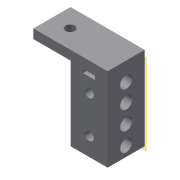
# Autodesk Inventor part: Neje_20mm_rod_connector_double
Saved by Autodesk Inventor 2019.4 (Build 234330000, 330)
## iProperties
Created: 2021-09-21
Part Number: Neje_20mm_rod_connector_double
Material: Generic
Document SubType Name: Modeling
Designer: diederichbenedict
Density: 1 g/cm^3
Appearance: Default
Author: diederichbenedict
Autodesk Inventor part; units mm, degrees
ref_plane "YZ Plane" through (0, 0, 0) normal (1, 0, 0) x (0, 1, 0)
ref_plane "XZ Plane" through (0, 0, 0) normal (0, 1, 0) x (-1, 0, 0)
ref_plane "Work Plane1" through (0, 0, 0) normal (0, 0, 1) x (1, 0, 0)
sketch "Sketch1" plane through (0, 0, 0) normal (0, 0, 1) x (1, 0, 0)
  circle A0 centre (0, 0) radius 2 construction
  circle A1 centre (0, 20) radius 2.5 construction
  line L0 (-10, 4) -> (-10, 16) construction
  line L1 (-10, 4) -> (-6, 4) construction
  line L2 (-6, 4) -> (-6, -4) construction
  line L3 (-6, -4) -> (-10, -4) construction
  line L4 (-10, -4) -> (-10, -10) construction
  line L5 (-10, -10) -> (-4, -10) construction
  line L6 (-4, -10) -> (-4, -6) construction
  line L7 (-4, -6) -> (4, -6) construction
  line L8 (4, -6) -> (4, -10) construction
  line L9 (4, -10) -> (10, -10) construction
  line L10 (10, -10) -> (10, -4) construction
  line L11 (10, -4) -> (6, -4) construction
  line L12 (6, -4) -> (6, 4) construction
  line L13 (6, 4) -> (10, 4) construction
  line L14 (10, 4) -> (10, 16) construction
  line L15 (6, 16) -> (10, 16) construction
  line L16 (6, 24) -> (6, 16) construction
  line L17 (10, 24) -> (6, 24) construction
  line L18 (10, 30) -> (10, 24) construction
  line L19 (4, 30) -> (10, 30) construction
  line L20 (4, 26) -> (4, 30) construction
  line L21 (-4, 26) -> (4, 26) construction
  line L22 (-4, 30) -> (-4, 26) construction
  line L23 (-10, 30) -> (-4, 30) construction
  line L24 (-10, 24) -> (-10, 30) construction
  line L25 (-6, 24) -> (-10, 24) construction
  line L26 (-6, 16) -> (-6, 24) construction
  line L27 (-10, 16) -> (-6, 16) construction
  line L28 (-4, 6) -> (-4, 14) construction
  line L29 (4, 14) -> (-4, 14) construction
  line L30 (4, 6) -> (4, 14) construction
  line L31 (4, 6) -> (-4, 6) construction
  line L32 (10, 30) -> (-10, 30)
  line L33 (-10, 30) -> (-10, -10)
  line L34 (-10, -10) -> (10, -10)
  line L35 (10, -10) -> (10, 30)
  circle A2 centre (0, 20) radius 2.5
  circle A3 centre (0, 0) radius 2.5
  point P0 (0, 0)
  dimension "d0" = 40
  dimension "d1" = 5
  constraints: 8 end point, 2 centre point, 2 coincident, 2 parallel, 1 concentric, 1 horizontal, 1 perpendicular
  measures "d0" distance of L33.end L32.end
  measures "d1" diameter of A3
ref_plane "Work Plane2" through (-30, -220, 20) normal (0, 0, 1) x (1, 0, 0)
extrude "Extrusion1" add sketch "Sketch1" along normal up to surface (20 mm away)
sketch "Sketch2" plane through (10, -10, 0) normal (1, 0, 0) x (0, 0, -1)
  line L0 (-20, 40) -> (-20, 0) projected
  line L1 (0, 0) -> (-20, 0) projected
  line L2 (0, 0) -> (0, 40) projected
  line L3 (0, 40) -> (-20, 40) projected
  line L4 (-14, 40) -> (-14, -210) projected
  line L5 (-6, 40) -> (-6, -210) projected
  line L6 (-20, 32.5) -> (-20, 27.5) projected
  line L7 (0, 32.5) -> (0, 27.5) projected
  line L8 (-20, 12.5) -> (-20, 7.5) projected
  line L9 (0, 12.5) -> (-20, 12.5) projected
  line L10 (0, 7.5) -> (-20, 7.5) projected
  line L11 (0, 32.5) -> (-20, 32.5) projected
  line L12 (0, 27.5) -> (-20, 27.5) projected
  circle A0 centre (-10, 45) radius 1.4
  circle A1 centre (-10, 25.349) radius 1.4
  circle A2 centre (-10, 15.349) radius 1.4
  circle A3 centre (-10, 35) radius 1.4
  circle A4 centre (-10, 5.349) radius 1.4
  point P0 (0, 10)
  point P1 (-9.8573, 5.349)
  dimension "d5" = 2.8
  dimension "d8" = 10
  dimension "d13" = 2.8
  dimension "d14" = 10
  constraints: 5 centre point, 1 vertical, 4 other
  measures "d5" diameter of A1
  measures "d8" distance of A1.centre A2.centre
  measures "d13" diameter of A4
  measures "d14" distance of A4.centre A2.centre
hole "Hole1" at (10, 25, 10) at (10, 5.349, 10) at (10, -4.651, 10) at (10, 15.349, 10) direction (-1, 0, 0) diameter 2.8 end through all counterbore diameter 6.5 counterbore depth 7
sketch "Sketch3" plane through (-10, 30, 0) normal (0, 1, 0) x (1, 0, 0)
  line L0 (0, -20) -> (20, -20) projected
  line L1 (20, 0) -> (20, -20) projected
  line L2 (20, 0) -> (0, 0) projected
  line L3 (0, 0) -> (0, -20) projected
  line L4 (20, 0) -> (0, 0) projected
  line L5 (20, 0) -> (-20, 0)
  line L6 (-20, 0) -> (-20, -20)
  line L7 (-20, -20) -> (20, -20)
  line L8 (20, -20) -> (20, 0)
  circle A0 centre (-10.1547, -10) radius 2.5
  point P0 (10, 0)
  dimension "d22" = 40
  dimension "d23" = 5
  constraints: 8 end point, 2 parallel, 1 centre point, 1 horizontal, 1 perpendicular
  measures "d22" distance of L7.end L6.end
  measures "d23" diameter of A0
extrude "Extrusion2" add sketch "Sketch3" along normal blind 5
sketch "Sketch5" plane through (-10, -10, 20) normal (0, 0, 1) x (1, 0, 0)
  line L0 (6.75, 39.4711) -> (13.25, 39.4711)
  line L1 (13.25, 39.4711) -> (13.25, 37.4711)
  line L2 (13.25, 37.4711) -> (6.75, 37.4711)
  line L3 (6.75, 37.4711) -> (6.75, 39.4711)
  line L4 (6.75, 39.4711) -> (13.25, 37.4711) construction
  line L5 (13.25, 39.4711) -> (6.75, 37.4711) construction
  point P0 (10, 10)
  point P1 (10, 38.4711)
  dimension "d33" = 6.5
  dimension "d34" = 2
  constraints: 12 end point, 2 midpoint, 2 parallel, 1 horizontal, 1 perpendicular
  measures "d33" distance of L1.end L2.end
  measures "d34" distance of L0.end L1.end
extrude "Extrusion3" cut sketch "Sketch5" against normal through all
body "Solid1"
